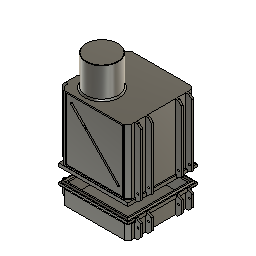
Outdoors Test Enclosure (Autodesk Fusion 360 design; units mm, degrees)
Autodesk Fusion 360 part; units mm, degrees
sketch "Sockets for components" plane through (0, 0, 0) normal (0, 0, 1) x (1, 0, 0)
  line L0 (0, 0) -> (100, 0)
  line L1 (100, 0) -> (100, 100)
  line L2 (100, 100) -> (0, 100)
  line L3 (0, 100) -> (0, 0)
  line L4 (5, 5) -> (56, 5)
  line L5 (56, 5) -> (56, 56)
  line L6 (56, 56) -> (5, 56)
  line L7 (5, 56) -> (5, 5)
  line L8 (95, 5) -> (75, 5)
  line L9 (75, 5) -> (75, 95)
  line L10 (75, 95) -> (95, 95)
  line L11 (95, 95) -> (95, 5)
  line L12 (5, 95) -> (70, 95)
  line L13 (70, 95) -> (70, 70)
  line L14 (70, 70) -> (5, 70)
  line L15 (5, 70) -> (5, 95)
  circle A0 centre (30.5, 30.4523) radius 22.5
  dimension "d1" = 100
  dimension "d2" = 100
  dimension "d3" = 51
  dimension "d4" = 51
  dimension "d5" = 20
  dimension "d6" = 90
  dimension "d7" = 65
  dimension "d8" = 25
  dimension "d9" = 45
  constraint horizontal L0
  constraint vertical L1
  constraint horizontal L2
  constraint vertical L3
  constraint coincident L0.start L3.end
  constraint horizontal L4
  constraint vertical L5
  constraint horizontal L6
  constraint vertical L7
  constraint horizontal L8
  constraint vertical L9
  constraint horizontal L10
  constraint vertical L11
  constraint horizontal L12
  constraint vertical L13
  constraint horizontal L14
  constraint vertical L15
  measures "d1" distance of L0.start L0.end
  measures "d2" distance of L0.start L2.end
  measures "d3" distance of L4.start L4.end
  measures "d4" distance of L4.start L6.end
  measures "d5" distance of L8.start L8.end
  measures "d6" distance of L8.start L10.end
  measures "d7" distance of L12.start L12.end
  measures "d8" distance of L12.start L14.end
  measures "d9" diameter of A0
extrude "Extrude1" add sketch "Sockets for components" along normal blind 103 contours L0 L1 L2 L3 | L4 L5 L6 L7 | L8 L9 L10 L11 | L12 L13 L14 L15 | A0 makes body 1
extrude "Extrude2" cut sketch "Sockets for components" along normal blind 49 contours L4 L5 L6 L7 | A0 bodies 1
extrude "Extrude3" cut sketch "Sockets for components" along normal blind 98 contours A0 bodies 1
extrude "Extrude4" cut sketch "Sockets for components" along normal blind 98 contours L12 L13 L14 L15 bodies 1
extrude "Extrude5" cut sketch "Sockets for components" along normal blind 98 contours L8 L9 L10 L11 bodies 1
extrude "Extrude6" add sketch "Sockets for components" against normal blind 25 from surface at -20 separate body contours L0 L1 L2 L3 | L4 L5 L6 L7 | L8 L9 L10 L11 | L12 L13 L14 L15 | A0 makes body 2
sketch "Enclosure base" plane through (0, 0, 0) normal (0, 0, 1) x (1, 0, 0)
  line L0 (5, 5) -> (95, 5)
  line L1 (95, 5) -> (95, 95)
  line L2 (95, 95) -> (5, 95)
  line L3 (5, 95) -> (5, 5)
  point P0 (5, 5)
  point P1 (95, 95)
  constraint horizontal L0
  constraint vertical L1
  constraint horizontal L2
  constraint vertical L3
  constraint coincident P1 L1.end
  constraint coincident P0 L0.start
extrude "Extrude7" cut sketch "Enclosure base" against normal blind 20 from surface at -20 bodies 2
sketch "Seal and outer edge" plane through (0, 0, 0) normal (0, 0, 1) x (1, 0, 0)
  line L0 (-2, -2) -> (102, -2)
  line L1 (102, -2) -> (102, 102)
  line L2 (102, 102) -> (-2, 102)
  line L3 (-2, 102) -> (-2, -2)
  line L4 (-0.5009, -0.4782) -> (100.4493, -0.4782)
  line L5 (100.4493, -0.4782) -> (100.4493, 100.4927)
  line L6 (100.4493, 100.4927) -> (-0.5009, 100.4927)
  line L7 (-0.5009, 100.4927) -> (-0.5009, -0.4782)
  line L8 (2.5379, 2.5762) -> (97.5094, 2.5762)
  line L9 (97.5094, 2.5762) -> (97.5094, 97.5266)
  line L10 (97.5094, 97.5266) -> (2.5379, 97.5266)
  line L11 (2.5379, 97.5266) -> (2.5379, 2.5762)
  constraint horizontal L0
  constraint vertical L1
  constraint horizontal L2
  constraint vertical L3
  constraint horizontal L4
  constraint vertical L5
  constraint horizontal L6
  constraint vertical L7
  constraint horizontal L8
  constraint vertical L9
  constraint horizontal L10
  constraint vertical L11
extrude "Extrude8" add sketch "Seal and outer edge" along normal blind 5 contours L0 L1 L2 L3 | L4 L5 L6 L7 bodies 1
extrude "Extrude9" add sketch "Seal and outer edge" against normal blind 5 from surface at -20 contours L0 L1 L2 L3 | L4 L5 L6 L7 bodies 2
extrude "Extrude10" cut sketch "Seal and outer edge" along normal blind 2.5 contours L4 L5 L6 L7 bodies 1
extrude "Extrude11" add sketch "Seal and outer edge" along normal blind 2 from surface at -20 contours L4 L5 L6 L7 bodies 2
chamfer "Chamfer1" distance 1.5 angle 53 1 faces at (34.1621, 0.5399, -18) on bodies 2
box "BoxPrimitive1" add length 98 width 3 height -9 placed x (0, 0, 1) y (0, -1, 0) z (1, 0, 0) at (0, 13, 5) bodies 1
box "BoxPrimitive2" add length 98 width 3 height 9 placed x (0, 0, 1) y (0, 1, 0) z (-1, 0, 0) at (0, 26, 5) bodies 1
box "BoxPrimitive3" add length 98 width 3 height 9 placed x (0, 0, 1) y (0, 1, 0) z (-1, 0, 0) at (0, 87, 5) bodies 1
box "BoxPrimitive4" add length 98 width 3 height 9 placed x (0, 0, 1) y (0, 1, 0) z (-1, 0, 0) at (0, 71, 5) bodies 1
box "BoxPrimitive5" add length 20 width 3 height 9 placed x (0, 0, -1) y (0, -1, 0) z (-1, 0, 0) at (0, 13, -25) bodies 2
box "BoxPrimitive8" add length 20 width 3 height 9 placed x (0, 0, -1) y (0, -1, 0) z (-1, 0, 0) at (0, 74, -25) bodies 2
box "BoxPrimitive9" add length 20 width 3 height 9 placed x (0, 0, -1) y (0, -1, 0) z (-1, 0, 0) at (0, 29, -25) bodies 2
box "BoxPrimitive10" add length 20 width 3 height 9 placed x (0, 0, -1) y (0, -1, 0) z (-1, 0, 0) at (0, 90, -25) bodies 2
box "BoxPrimitive11" add length 98 width 3 height 9 placed x (0, 0, 1) y (0, -1, 0) z (1, 0, 0) at (100, 90, 5) bodies 1
box "BoxPrimitive12" add length 98 width 3 height 9 placed x (0, 0, 1) y (0, -1, 0) z (1, 0, 0) at (100, 74, 5) bodies 1
box "BoxPrimitive13" add length 98 width 3 height 9 placed x (0, 0, 1) y (0, -1, 0) z (1, 0, 0) at (100, 13, 5) bodies 1
box "BoxPrimitive14" add length 98 width 3 height 9 placed x (0, 0, 1) y (0, -1, 0) z (1, 0, 0) at (100, 29, 5) bodies 1
box "BoxPrimitive15" add length 20 width 3 height 9 placed x (0, 0, -1) y (0, 1, 0) z (1, 0, 0) at (100, 87, -25) bodies 2
box "BoxPrimitive16" add length 20 width 3 height 9 placed x (0, 0, -1) y (0, 1, 0) z (1, 0, 0) at (100, 71, -25) bodies 2
box "BoxPrimitive17" add length 20 width 3 height 9 placed x (0, 0, -1) y (0, 1, 0) z (1, 0, 0) at (100, 10, -25) bodies 2
box "BoxPrimitive18" add length 20 width 3 height 9 placed x (0, 0, -1) y (0, 1, 0) z (1, 0, 0) at (100, 26, -25) bodies 2
chamfer "Chamfer2" distance 5 angle 45 8 edges at (-9, 11.5, -45) (-9, 27.5, -45) (-9, 72.5, -45) (-9, 88.5, -45) (109, 11.5, -45) (109, 27.5, -45) (109, 72.5, -45) (109, 88.5, -45) measured on face at (-9, 11, -31.6667) measured on face at (-9, 27, -31.6667) measured on face at (-9, 72, -31.6667) measured on face at (-9, 88, -31.6667) measured on face at (109, 12, -31.6667) measured on face at (109, 28, -31.6667) measured on face at (109, 73, -31.6667) measured on face at (109, 89, -31.6667) on bodies 2
chamfer "Chamfer3" distance 5 angle 45 8 edges at (109, 88.5, 103) (109, 72.5, 103) (109, 27.5, 103) (109, 11.5, 103) (-9, 11.5, 103) (-9, 27.5, 103) (-9, 72.5, 103) (-9, 88.5, 103) measured on face at (109, 88, 37.6667) measured on face at (109, 72, 37.6667) measured on face at (109, 27, 37.6667) measured on face at (109, 11, 37.6667) measured on face at (-9, 11, 37.6667) measured on face at (-9, 28, 37.6667) measured on face at (-9, 73, 37.6667) measured on face at (-9, 89, 37.6667) on bodies 1
chamfer "Chamfer4" distance 5 angle 45 8 edges at (0, 0, -35) (100, 0, -35) (0, 100, -35) (100, 100, -35) (0, 100, 54) (100, 100, 54) (0, 0, 54) (100, 0, 54) measured on face at (33.3333, 0, -31.6667) measured on face at (100, 3.3333, -38.3333) measured on face at (0, 96.6667, -31.6667) measured on face at (66.6667, 100, -31.6667) measured on face at (66.6667, 100, 37.6667) measured on face at (100, 93.3333, 70.3333) measured on face at (0, 6.6667, 70.3333) measured on face at (33.3333, 0, 37.6667) on bodies 1 2
sketch "Hinge holes" plane through (0, 100, 0) normal (0, 1, 0) x (-1, 0, 0)
  line L0 (-95, 103) -> (-95, 5)
  line L1 (-95, 5) -> (-5, 5)
  line L2 (-5, 5) -> (-5, 103)
  line L3 (-5, 103) -> (-95, 103)
  line L4 (9, 0) -> (5, 0)
  line L5 (5, 0) -> (5, 12)
  line L6 (5, 12) -> (9, 12)
  line L7 (9, 12) -> (9, 0)
  line L8 (9, -20) -> (5, -20)
  line L9 (5, -20) -> (5, -32)
  line L10 (5, -32) -> (9, -32)
  line L11 (9, -32) -> (9, -20)
  line L12 (-109, 0) -> (-105, 0)
  line L13 (-105, 0) -> (-105, 12)
  line L14 (-105, 12) -> (-109, 12)
  line L15 (-109, 12) -> (-109, 0)
  line L16 (-109, -20) -> (-105, -20)
  line L17 (-105, -20) -> (-105, -32)
  line L18 (-105, -32) -> (-109, -32)
  line L19 (-109, -32) -> (-109, -20)
  dimension "d161" = 12
  dimension "d162" = 4
  dimension "d163" = 12
  dimension "d164" = 4
  dimension "d165" = 12
  dimension "d166" = 4
  dimension "d167" = 12
  constraint horizontal L4
  constraint vertical L5
  constraint horizontal L6
  constraint vertical L7
  constraint horizontal L8
  constraint vertical L9
  constraint horizontal L10
  constraint vertical L11
  constraint horizontal L12
  constraint vertical L13
  constraint horizontal L14
  constraint vertical L15
  constraint horizontal L16
  constraint vertical L17
  constraint horizontal L18
  constraint vertical L19
  measures "d161" distance of L4.start L6.end
  measures "d162" distance of L8.start L8.end
  measures "d163" distance of L8.start L10.end
  measures "d164" distance of L12.start L12.end
  measures "d165" distance of L12.start L14.end
  measures "d166" distance of L16.start L16.end
  measures "d167" distance of L16.start L18.end
hole "Hole4" at (-5, 100, -32) at (-5, 100, 12) at (105, 100, 12) at (105, 100, -32) direction (0, -1, 0) diameter 3 depth 90 tip angle 118 bodies 1 2
chamfer "Chamfer5" distance 7 angle 30 8 edges at (102, 11.5, 5) (102, 27.5, 5) (102, 72.5, 5) (102, 88.5, 5) (102, 11.5, -25) (102, 27.5, -25) (102, 72.5, -25) (102, 88.5, -25) measured on face at (104.3333, 12, 5) measured on face at (104.3333, 28, 5) measured on face at (104.3333, 73, 5) measured on face at (104.3333, 89, 5) measured on face at (106.6667, 12, -25) measured on face at (106.6667, 28, -25) measured on face at (106.6667, 73, -25) measured on face at (106.6667, 89, -25) on bodies 1 2
chamfer "Chamfer6" distance 7 angle 30 8 edges at (-2, 27.5, 5) (-2, 11.5, 5) (-2, 72.5, 5) (-2, 88.5, 5) (-2, 88.5, -25) (-2, 72.5, -25) (-2, 27.5, -25) (-2, 11.5, -25) measured on face at (-4.3333, 27, 5) measured on face at (-6.6667, 12, 5) measured on face at (-4.3333, 72, 5) measured on face at (-4.3333, 88, 5) measured on face at (-4.3333, 89, -25) measured on face at (-4.3333, 73, -25) measured on face at (-4.3333, 28, -25) measured on face at (-4.3333, 12, -25) on bodies 1 2
sketch "Radiator plate edge" plane through (0, 0, 0) normal (0, 1, 0) x (1, 0, 0)
  line L0 (5, -103) -> (95, -103)
  line L1 (95, -103) -> (95, -5)
  line L2 (95, -5) -> (5, -5)
  line L3 (5, -5) -> (5, -103)
  line L4 (7, -101) -> (93, -101)
  line L5 (93, -101) -> (93, -7)
  line L6 (93, -7) -> (7, -7)
  line L7 (7, -7) -> (7, -101)
  constraint horizontal L0
  constraint vertical L1
  constraint horizontal L2
  constraint vertical L3
  constraint horizontal L4
  constraint vertical L5
  constraint horizontal L6
  constraint vertical L7
extrude "Extrude12" add sketch "Radiator plate edge" against normal blind 1.5 bodies 1
extrude "Extrude13" add 9 faces at (-1.3333, 89, -45) (-1.3333, 73, -45) (-1.3333, 12, -45) (-1.3333, 28, -45) (66.6667, 43, -45) (101.3333, 88, -45) (101.3333, 11, -45) (101.3333, 72, -45) (101.3333, 27, -45) along direction (0, 0, -1) blind 3 on bodies 2 bodies 2
box "BoxPrimitive19" add length 78 width 13 height 9 placed x (0, 0, 1) y (0, 1, 0) z (-1, 0, 0) at (0, 74, 20) bodies 1
box "BoxPrimitive20" add length 78 width 13 height 9 placed x (0, 0, -1) y (0, -1, 0) z (-1, 0, 0) at (0, 26, 98) bodies 1
extrude "Extrude14" add 1 faces at (-4.3333, 13, 99.6667) along direction (0, 1, 0) blind 13 on bodies 1 bodies 1
extrude "Extrude15" add 1 faces at (-4.3333, 74, 99.6667) along direction (0, 1, 0) blind 13 on bodies 1 bodies 1
extrude "Extrude16" add 2 faces at (-3, 21.6667, 20) (-3, 78.3333, 20) along direction (0, 0, -1) blind 3 on bodies 1 bodies 1
sketch "Vesa mount hole placement" plane through (-9, 0, 0) normal (-1, 0, 0) x (0, -1, 0)
  line L0 (-10, 98) -> (-29, 98)
  line L1 (-29, 98) -> (-29, 5)
  line L2 (-29, 5) -> (-26, 5)
  line L3 (-26, 5) -> (-26, 17)
  line L4 (-26, 17) -> (-13, 17)
  line L5 (-13, 17) -> (-13, 5)
  line L6 (-13, 5) -> (-10, 5)
  line L7 (-10, 5) -> (-10, 98)
  line L8 (-12.5, 20.5) -> (-87.5, 20.5)
  line L9 (-87.5, 20.5) -> (-87.5, 95.5)
  line L10 (-87.5, 95.5) -> (-12.5, 95.5)
  line L11 (-12.5, 95.5) -> (-12.5, 20.5)
  line L12 (-25, 33) -> (-75, 33)
  line L13 (-75, 33) -> (-75, 83)
  line L14 (-75, 83) -> (-25, 83)
  line L15 (-25, 83) -> (-25, 33)
  dimension "d215" = 75
  dimension "d216" = 75
  dimension "d217" = 50
  dimension "d218" = 50
  constraint horizontal L8
  constraint vertical L9
  constraint horizontal L10
  constraint vertical L11
  constraint horizontal L12
  constraint vertical L13
  constraint horizontal L14
  constraint vertical L15
  measures "d215" distance of L8.start L8.end
  measures "d216" distance of L8.start L10.end
  measures "d217" distance of L12.start L12.end
  measures "d218" distance of L12.start L14.end
hole "Hole5" at (-9, 12.5, 20.5) at (-9, 12.5, 95.5) at (-9, 87.5, 20.5) at (-9, 87.5, 95.5) at (-9, 75, 83) at (-9, 75, 33) at (-9, 25, 33) at (-9, 25, 83) direction (1, 0, 0) diameter 3.75 depth 4 tip angle 180 bodies 1
sketch "Lid vesa mount" plane through (0, 0, -48) normal (0, 0, -1) x (1, 0, 0)
  line L0 (95, -100) -> (100, -95)
  line L1 (100, -95) -> (100, -90)
  line L2 (100, -90) -> (104, -90)
  line L3 (104, -90) -> (104, -87)
  line L4 (104, -87) -> (100, -87)
  line L5 (100, -87) -> (100, -74)
  line L6 (100, -74) -> (104, -74)
  line L7 (104, -74) -> (104, -71)
  line L8 (104, -71) -> (100, -71)
  line L9 (100, -71) -> (100, -29)
  line L10 (100, -29) -> (104, -29)
  line L11 (104, -29) -> (104, -26)
  line L12 (104, -26) -> (100, -26)
  line L13 (100, -26) -> (100, -13)
  line L14 (100, -13) -> (104, -13)
  line L15 (104, -13) -> (104, -10)
  line L16 (104, -10) -> (100, -10)
  line L17 (100, -10) -> (100, -5)
  line L18 (100, -5) -> (95, 0)
  line L19 (95, 0) -> (5, 0)
  line L20 (5, 0) -> (0, -5)
  line L21 (0, -5) -> (0, -10)
  line L22 (0, -10) -> (-4, -10)
  line L23 (-4, -10) -> (-4, -13)
  line L24 (-4, -13) -> (0, -13)
  line L25 (0, -13) -> (0, -26)
  line L26 (0, -26) -> (-4, -26)
  line L27 (-4, -26) -> (-4, -29)
  line L28 (-4, -29) -> (0, -29)
  line L29 (0, -29) -> (0, -71)
  line L30 (0, -71) -> (-4, -71)
  line L31 (-4, -71) -> (-4, -74)
  line L32 (-4, -74) -> (0, -74)
  line L33 (0, -74) -> (0, -87)
  line L34 (0, -87) -> (-4, -87)
  line L35 (-4, -87) -> (-4, -90)
  line L36 (-4, -90) -> (0, -90)
  line L37 (0, -90) -> (0, -95)
  line L38 (0, -95) -> (5, -100)
  line L39 (5, -100) -> (95, -100)
  line L40 (2.5, -97.5) -> (2.5, -2.5)
  line L41 (2.5, -2.5) -> (97.5, -2.5)
  line L42 (87.5, -87.5) -> (12.5, -87.5)
  line L43 (12.5, -87.5) -> (12.5, -12.5)
  line L44 (12.5, -12.5) -> (87.5, -12.5)
  line L45 (87.5, -12.5) -> (87.5, -87.5)
  line L46 (75, -75) -> (25, -75)
  line L47 (25, -75) -> (25, -25)
  line L48 (25, -25) -> (75, -25)
  line L49 (75, -25) -> (75, -75)
  dimension "d226" = 75
  dimension "d227" = 75
  dimension "d228" = 50
  dimension "d229" = 50
  constraint vertical L40
  constraint horizontal L41
  constraint midpoint L20 L40.end
  constraint horizontal L42
  constraint vertical L43
  constraint horizontal L44
  constraint vertical L45
  constraint horizontal L46
  constraint vertical L47
  constraint horizontal L48
  constraint vertical L49
  measures "d226" distance of L42.start L42.end
  measures "d227" distance of L42.start L44.end
  measures "d228" distance of L46.start L46.end
  measures "d229" distance of L46.start L48.end
hole "Hole6" at (25, 25, -48) at (12.5, 12.5, -48) at (87.5, 87.5, -48) at (75, 75, -48) at (25, 75, -48) at (12.5, 87.5, -48) at (75, 25, -48) at (87.5, 12.5, -48) direction (0, 0, 1) diameter 3.75 depth 4 tip angle 180 bodies 2
extrude "Extrude17" add 4 faces at (-4, 89, -46) (-4, 73, -46) (-4, 28, -46) (-4, 12, -46) along direction (-1, 0, 0) blind 5 on bodies 2 bodies 2
extrude "Extrude18" add 4 faces at (104, 88, -46) (104, 72, -46) (104, 27, -46) (104, 11, -46) along direction (1, 0, 0) blind 5 on bodies 2 bodies 2
extrude "Extrude19" add 4 faces at (-5.6667, 12, -45) (-5.6667, 28, -45) (-5.6667, 73, -45) (-5.6667, 89, -45) along direction (0, 0, 1) blind 5 on bodies 2 bodies 2
extrude "Extrude20" add 4 faces at (105.6667, 88, -45) (105.6667, 72, -45) (105.6667, 27, -45) (105.6667, 11, -45) along direction (0, 0, 1) blind 5 on bodies 2 bodies 2
chamfer "Chamfer7" distance 5 angle 45 8 edges at (109, 88.5, -48) (109, 72.5, -48) (109, 27.5, -48) (109, 11.5, -48) (-9, 27.5, -48) (-9, 11.5, -48) (-9, 72.5, -48) (-9, 88.5, -48) measured on face at (109, 89, -40.3333) measured on face at (109, 72, -32.6667) measured on face at (109, 27, -32.6667) measured on face at (109, 11, -32.6667) measured on face at (-9, 28, -32.6667) measured on face at (-9, 12, -32.6667) measured on face at (-9, 73, -32.6667) measured on face at (-9, 89, -32.6667) on bodies 2
chamfer "Chamfer8" distance 1 angle 60 2 faces at (99, 1, -25) (99, 99, -25) on bodies 2
chamfer "Chamfer9" distance 1 angle 45 1 faces at (99, 99, 5) on bodies 1
chamfer "Chamfer10" distance 1 angle 45 2 edges at (97.5, 2.5, 5) (2.5, 2.5, 5) measured on face at (98.3333, 3.3333, 37.6667) measured on face at (3.3333, 1.6667, 37.6667) on bodies 1
extrude "Extrude21" cut sketch "Sockets for components" along normal blind 98 contours L4 L5 L6 L7 | A0 bodies 1
sketch "Scintillator enclosure cylinder" plane through (0, 0, 0) normal (0, 0, 1) x (1, 0, 0)
  circle A0 centre (30.5, 30.4523) radius 24
  point P0 (30.5, 30.4523)
  dimension "d257" = 48
  constraint coincident P0 A0.centre
  measures "d257" diameter of A0
extrude "Extrude22" add sketch "Scintillator enclosure cylinder" along normal blind 51 from surface at 98 bodies 1
extrude "Extrude23" cut sketch "Sockets for components" along normal blind 49 from surface at 98 contours A0 bodies 1
chamfer "Chamfer11" distance 2 angle 45 1 edges at (8.1241, 39.131, 103) on bodies 1
sketch "Heat pipe interfacing" plane through (0, 0, 0) normal (0, 1, 0) x (1, 0, 0)
  line L0 (21, -78) -> (0, -78)
  line L1 (0, -78) -> (0, -103)
  line L2 (0, -103) -> (21, -103)
  line L3 (21, -103) -> (21, -78)
  line L4 (19.4, -75) -> (19.4, -81)
  arc A0 (19.4, -81) -> (22.6, -81) centre (21, -81) ccw
  line L5 (22.6, -81) -> (22.6, -75)
  arc A1 (22.6, -75) -> (19.4, -75) centre (21, -75) ccw
  line L6 (21, -75) -> (21, -81) construction
  line L7 (21, -82.6) -> (66.9039, -82.6)
  line L8 (66.9039, -82.6) -> (66.9039, -73.4)
  line L9 (66.9039, -73.4) -> (21, -73.4)
  line L10 (21, -73.4) -> (21, -82.6)
  line L11 (15, -90) -> (86.5335, -17.2885)
  line L12 (32.4085, -69.8095) -> (13.7525, -88.7727)
  arc A2 (13.7525, -88.7727) -> (16.2475, -91.2273) centre (15, -90) ccw
  line L13 (16.2475, -91.2273) -> (34.9035, -72.2641)
  arc A3 (34.9035, -72.2641) -> (32.4085, -69.8095) centre (33.656, -71.0368) ccw
  line L14 (33.656, -71.0368) -> (15, -90) construction
  point P0 (21, -78)
  point P1 (24.328, -80.5184)
  dimension "d265" = 21
  dimension "d266" = 25
  dimension "d267" = 3.2
  dimension "d287" = 102
  dimension "d298" = 3.5
  constraint horizontal L0
  constraint vertical L1
  constraint horizontal L2
  constraint vertical L3
  constraint tangent L4 A0
  constraint tangent A0 L5
  constraint parallel L4 L5
  constraint tangent L5 A1
  constraint tangent L4 A1
  constraint coincident L3 A0.centre
  constraint perpendicular L0 L6
  constraint coincident P0 L0.start
  constraint midpoint L6 P0
  constraint horizontal L7
  constraint vertical L8
  constraint horizontal L9
  constraint vertical L10
  constraint midpoint A0 L7.start
  constraint tangent L12 A2
  constraint tangent A2 L13
  constraint parallel L12 L13
  constraint tangent L13 A3
  constraint tangent L12 A3
  constraint coincident L11.start A2.centre
  constraint parallel L11 L14
  constraint coincident L11 P1
  constraint midpoint L14 P1
  measures "d265" distance of P0 L0.end
  measures "d266" distance of P0 L2.end
  measures "d267" diameter of A0
  measures "d287" distance of L11.start L11.end
  measures "d298" diameter of A2
sketch "Rosspad with metal plate" plane through (0, 0, 0) normal (0, 0, 1) x (1, 0, 0)
  line L0 (56, 56) -> (5, 56)
  line L1 (5, 56) -> (5, 4)
  line L2 (5, 4) -> (56, 4)
  line L3 (56, 4) -> (56, 56)
  point P0 (56, 56)
  dimension "d284" = 52
  constraint horizontal L0
  constraint vertical L1
  constraint horizontal L2
  constraint vertical L3
  constraint coincident P0 L0.start
  measures "d284" distance of P0 L2.end
extrude "Extrude28" cut sketch "Rosspad with metal plate" along normal blind 98 bodies 1
pipe "Pipe3" cut diameter 3.2 path "Heat pipe interfacing" along L11 bodies 1
fillet "Fillet9" radius 1 2 edges at (15, 1.6, 90) (86.5335, 1.6, 17.2885) on bodies 1
extrude "Extrude29" cut sketch "Heat pipe interfacing" along normal blind 6 contours L3 A0 L5 L10 L12 | L3 A0 L10 L12 | L3 L7 L11 | L3 A0 L12 A2 L13 | A0 L5 L7 L9 L11 L12 | L9 L11 L12 A3 | L3 L7 L11 L13 | L7 L9 L11 L13 | L9 L11 L13 A3 bodies 1
fillet "Fillet10" radius 10 1 edges at (34.8833, 1.6, 69.7893) on bodies 1
chamfer "Chamfer12" distance 0.5 angle 45 1 edges at (8.1241, 21.7735, 149) on bodies 1
named bodies: "Enclosure body", "Enclosure lid"
